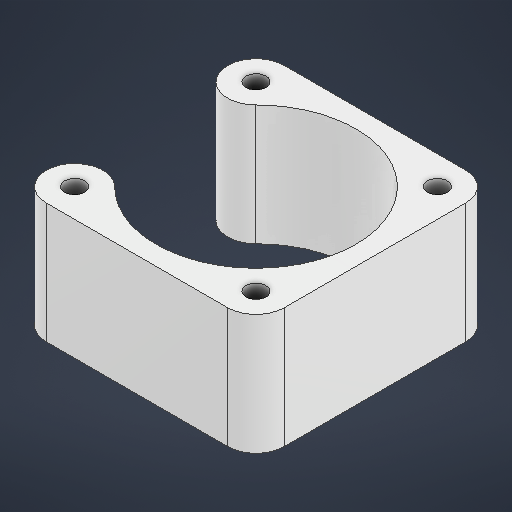
# Autodesk Inventor part: CNC-009-XAxisNema23Spacer
Saved by Autodesk Inventor 2026.2 (Build 302298000, 298)
## iProperties
Created: 2026-06-15
Part Number: CNC-009-XAxisNema23Spacer
Material: ABS Plastic
Document SubType Name: Modeling
Designer: Kenji
Density: 1.06 g/cm^3
Appearance: Smooth - White
Author: Kenji
Autodesk Inventor part; units mm, degrees
ref_plane "YZ Plane" through (0, 0, 0) normal (1, 0, 0) x (0, 1, 0)
ref_plane "XZ Plane" through (0, 0, 0) normal (0, 1, 0) x (-1, 0, 0)
ref_plane "XY Plane" through (0, 0, 0) normal (0, 0, 1) x (1, 0, 0)
sketch "Sketch1" plane through (0, 0, 0) normal (0, 1, 0) x (-1, 0, 0)
  circle A0 centre (0, 0) radius 8.0947
  circle A1 centre (23.57, 23.57) radius 2.6
  circle A2 centre (23.57, -23.57) radius 2.6
  circle A3 centre (-23.57, -23.57) radius 2.6
  circle A4 centre (-23.57, 23.57) radius 2.6
  circle A5 centre (23.57, 23.57) radius 7.3625 construction
  circle A6 centre (23.57, -23.57) radius 7.3625 construction
  circle A7 centre (-23.57, -23.57) radius 7.3625 construction
  circle A8 centre (-23.57, 23.57) radius 7.3625 construction
  line L0 (23.57, 30.9325) -> (-23.57, 30.9325)
  line L1 (-30.9325, 23.57) -> (-30.9325, -23.57)
  line L2 (-23.57, -30.9325) -> (23.57, -30.9325)
  arc A9 (18.3639, 18.3639) -> (23.57, 30.9325) centre (23.57, 23.57) ccw
  arc A10 (23.57, -30.9325) -> (18.3639, -18.3639) centre (23.57, -23.57) ccw
  circle A11 centre (0, 0) radius 25.9705 construction
  arc A12 (18.3639, 18.3639) -> (18.3639, -18.3639) centre (0, 0) ccw
  arc A13 (-23.57, 30.9325) -> (-30.9325, 23.57) centre (-23.57, 23.57) ccw
  arc A14 (-30.9325, -23.57) -> (-23.57, -30.9325) centre (-23.57, -23.57) ccw
  dimension "d0" = 16.1894
  dimension "d1" = 5.2
  dimension "d2" = 23.57
  dimension "d3" = 23.57
  dimension "d4" = 23.57
  dimension "d5" = 23.57
  dimension "d6" = 4.7625
  constraints: 20 point on circle, 15 centre point, 10 tangent, 8 equal radius, 6 end point, 5 coincident, 2 horizontal alignment, 2 vertical alignment, 1 horizontal
  measures "d0" diameter of A0
  measures "d1" diameter of A1
  measures "d2" horizontal distance of point (0, 0) A1.centre
  measures "d3" horizontal distance of point (0, 0) A1.centre
  measures "d4" horizontal distance of A3.centre point (0, 0)
  measures "d5" horizontal distance of A3.centre point (0, 0)
  measures "d6" radial gap between concentric circles of A5 A1
extrude "Extrusion1" add sketch "Sketch1" along normal blind 31.2375 contours A9 A12 A10 L2 A14 L1 A13 L0
body "Solid1"
